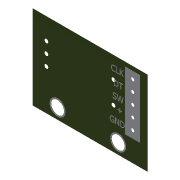
# Autodesk Inventor part: decal_encoder
Saved by Autodesk Inventor 2014 (Build 180170000, 170)
## iProperties
Created: 2015-11-19
Part Number: decal_encoder
Material: Generic
Document SubType Name: Modeling
Designer: Tom
Density: 1 g/cm^3
Appearance: Default
Autodesk Inventor part; units mm, degrees
ref_plane "YZ Plane" through (0, 0, 0) normal (1, 0, 0) x (0, 1, 0)
ref_plane "XZ Plane" through (0, 0, 0) normal (0, 1, 0) x (-1, 0, 0)
ref_plane "XY Plane" through (0, 0, 0) normal (0, 0, 1) x (1, 0, 0)
sketch "0" plane through (0, 0, 0) normal (0, 0, 1) x (1, 0, 0)
  line L0 (0, 0) -> (26.416, 0)
  line L1 (26.416, 0) -> (26.416, 19.3294)
  line L2 (26.416, 19.3294) -> (0, 19.3294)
  line L3 (0, 19.3294) -> (0, 0)
  circle A0 centre (3.175, 14.4018) radius 0.4445
  circle A1 centre (3.175, 11.8618) radius 0.4445
  circle A2 centre (3.175, 9.3218) radius 0.4445
  circle A3 centre (5.7658, 2.4638) radius 1.5
  circle A4 centre (19.685, 2.4638) radius 1.5
  circle A5 centre (23.0251, 6.5532) radius 0.381
  circle A6 centre (23.0251, 9.0932) radius 0.381
  circle A7 centre (23.0251, 11.6332) radius 0.381
  circle A8 centre (23.0251, 14.1732) radius 0.381
  circle A9 centre (23.0251, 16.7132) radius 0.381
  circle A10 centre (5.7658, 2.4638) radius 1.778
  circle A11 centre (19.685, 2.4638) radius 1.778
  line L4 (21.3741, 4.9022) -> (24.6761, 4.9022)
  line L5 (24.6761, 4.9022) -> (24.6761, 18.3642)
  line L6 (21.3741, 18.3642) -> (21.3741, 4.9022)
  circle A12 centre (23.0251, 16.7132) radius 0.4445 projected
  line L7 (24.6761, 18.3642) -> (21.3741, 18.3642)
  line L8 (18.8514, 15.1638) -> (18.8514, 13.6398) projected
  circle A13 centre (18.593, 14.4018) radius 0.4445 projected
  circle A14 centre (18.593, 9.3218) radius 0.4445 projected
  dimension "d0" = 3.556
  dimension "d1" = 3.556
  dimension "d3" = 13.462
  dimension "d4" = 10.16
  dimension "d5" = 13.462
  dimension "d7" = 2.54
  dimension "d8" = 2.54
  dimension "d9" = 2.54
  dimension "d10" = 2.54
  dimension "d11" = 1.651
  dimension "d26" = 0
  dimension "d27" = 2.54
  dimension "d28" = 2.54
  constraints: 16 end point, 12 centre point, 3 vertical alignment, 2 coincident, 2 perpendicular, 1 horizontal, 1 parallel
  measures "d0" diameter of A11
  measures "d1" diameter of A10
  measures "d3" distance of L6.start L4.start
  measures "d4" distance of A5.centre A9.centre
  measures "d5" distance of L5.end L4.end
  measures "d7" distance of A8.centre A9.centre
  measures "d8" distance of A7.centre A8.centre
  measures "d9" distance of A7.centre A6.centre
  measures "d10" distance of A5.centre A6.centre
  measures "d11" horizontal distance of L5.end A9.centre
  measures "d26" vertical distance of A0.centre A13.centre
  measures "d27" distance of A0.centre A1.centre
  measures "d28" distance of A2.centre A1.centre
extrude "Extrusion1" add sketch "0" along normal blind 0.0254 contours L3 L2 L1 L0 | A10 | A11 | L6 L7 L5 L4 | A12 | A13 L8 | L8 A13 | A14
sketch "Sketch3" plane through (0, 0, 0.0254) normal (0, 0, 1) x (1, 0, 0)
  circle A0 centre (23.0251, 16.7132) radius 0.381 projected
  circle A1 centre (23.0251, 14.1732) radius 0.381 projected
  circle A2 centre (23.0251, 11.6332) radius 0.381 projected
  circle A3 centre (23.0251, 9.0932) radius 0.381 projected
  circle A4 centre (23.0251, 6.5532) radius 0.381 projected
  circle A5 centre (19.685, 2.4638) radius 1.5 projected
  circle A6 centre (5.7658, 2.4638) radius 1.5 projected
  line L0 (21.3106, 18.3642) -> (24.7396, 18.3642)
  line L1 (24.7396, 18.3642) -> (24.7396, 4.9022)
  line L2 (24.7396, 4.9022) -> (21.3106, 4.9022)
  line L3 (21.3106, 4.9022) -> (21.3106, 18.3642)
  circle A7 centre (19.685, 2.4638) radius 1.8143
  circle A8 centre (5.7658, 2.4638) radius 1.8161
  line L4 (18.02, 17.393) -> (20.1128, 17.393) construction
  line L5 (20.1128, 17.393) -> (20.1128, 15.9127) construction
  line L6 (20.1128, 15.9127) -> (18.02, 15.9127) construction
  line L7 (18.02, 15.9127) -> (18.02, 17.393) construction
  line L8 (18.6153, 14.6193) -> (20.8208, 14.6193) construction
  line L9 (20.8208, 14.6193) -> (20.8208, 13.19) construction
  line L10 (20.8208, 13.19) -> (18.6153, 13.19) construction
  line L11 (18.6153, 13.19) -> (18.6153, 14.6193) construction
  line L12 (18.3939, 11.9822) -> (20.9411, 11.9822) construction
  line L13 (20.9411, 11.9822) -> (20.9411, 10.6669) construction
  line L14 (20.9411, 10.6669) -> (18.3939, 10.6669) construction
  line L15 (18.3939, 10.6669) -> (18.3939, 11.9822) construction
  line L16 (19.4486, 9.4797) -> (20.7196, 9.4797) construction
  line L17 (20.7196, 9.4797) -> (20.7196, 8.4824) construction
  line L18 (20.7196, 8.4824) -> (19.4486, 8.4824) construction
  line L19 (19.4486, 8.4824) -> (19.4486, 9.4797) construction
  line L20 (17.713, 7.1316) -> (21.2297, 7.1316) construction
  line L21 (21.2297, 7.1316) -> (21.2297, 5.8142) construction
  line L22 (21.2297, 5.8142) -> (17.713, 5.8142) construction
  line L23 (17.713, 5.8142) -> (17.713, 7.1316) construction
  spline S0 degree 2 poles (18.3738, 5.8142) (18.2389, 5.8142) (18.0156, 5.8966) (17.9353, 5.9799) knots 0 0 0 1 2 2 2
  spline S1 degree 2 poles (17.9353, 5.9799) (17.8551, 6.0643) (17.7696, 6.3134) (17.7696, 6.475) knots 0 0 0 1 2 2 2
  spline S2 degree 2 poles (17.7696, 6.475) (17.7696, 6.6283) (17.8561, 6.8712) (17.9364, 6.9576) knots 0 0 0 1 2 2 2
  spline S3 degree 2 poles (17.9364, 6.9576) (18.0135, 7.041) (18.24, 7.1316) (18.3748, 7.1316) knots 0 0 0 1 2 2 2
  spline S4 degree 2 poles (18.3748, 7.1316) (18.4396, 7.1316) (18.557, 7.113) (18.6105, 7.0966) knots 0 0 0 1 2 2 2
  spline S5 degree 2 poles (18.6105, 7.0966) (18.6537, 7.0842) (18.7587, 7.0389) (18.7906, 7.0225) knots 0 0 0 1 2 2 2
  line L24 (18.7906, 7.0225) -> (18.7906, 6.8187)
  line L25 (18.7906, 6.8187) -> (18.7762, 6.8187)
  spline S6 degree 2 poles (18.7762, 6.8187) (18.7443, 6.8465) (18.6774, 6.8969) (18.6156, 6.9257) knots 0 0 0 1 2 2 2
  spline S7 degree 2 poles (18.6156, 6.9257) (18.5642, 6.9515) (18.4314, 6.9854) (18.3552, 6.9854) knots 0 0 0 1 2 2 2
  spline S8 degree 2 poles (18.3552, 6.9854) (18.172, 6.9854) (17.9456, 6.7096) (17.9456, 6.4801) knots 0 0 0 1 2 2 2
  spline S9 degree 2 poles (17.9456, 6.4801) (17.9456, 6.3525) (18.0053, 6.1611) (18.0619, 6.0952) knots 0 0 0 1 2 2 2
  spline S10 degree 2 poles (18.0619, 6.0952) (18.1165, 6.0293) (18.2708, 5.9604) (18.3676, 5.9604) knots 0 0 0 1 2 2 2
  spline S11 degree 2 poles (18.3676, 5.9604) (18.4386, 5.9604) (18.5806, 5.981) (18.629, 6.0015) knots 0 0 0 1 2 2 2
  line L26 (18.629, 6.0015) -> (18.629, 6.3298)
  line L27 (18.629, 6.3298) -> (18.3347, 6.3298)
  line L28 (18.3347, 6.3298) -> (18.3347, 6.478)
  line L29 (18.3347, 6.478) -> (18.7957, 6.478)
  line L30 (18.7957, 6.478) -> (18.7957, 5.9233)
  spline S12 degree 2 poles (18.7957, 5.9233) (18.7638, 5.9089) (18.6547, 5.8647) (18.6084, 5.8513) knots 0 0 0 1 2 2 2
  spline S13 degree 2 poles (18.6084, 5.8513) (18.5456, 5.8328) (18.4448, 5.8142) (18.3738, 5.8142) knots 0 0 0 1 2 2 2
  line L31 (19.9165, 5.8389) -> (19.7271, 5.8389)
  line L32 (19.7271, 5.8389) -> (19.1652, 6.934)
  line L33 (19.1652, 6.934) -> (19.1652, 5.8389)
  line L34 (19.1652, 5.8389) -> (19.0077, 5.8389)
  line L35 (19.0077, 5.8389) -> (19.0077, 7.1089)
  line L36 (19.0077, 7.1089) -> (19.2475, 7.1089)
  line L37 (19.2475, 7.1089) -> (19.759, 6.1034)
  line L38 (19.759, 6.1034) -> (19.759, 7.1089)
  line L39 (19.759, 7.1089) -> (19.9165, 7.1089)
  line L40 (19.9165, 7.1089) -> (19.9165, 5.8389)
  spline S14 degree 2 poles (21.1752, 6.4729) (21.1752, 6.299) (21.0342, 6.019) (20.9158, 5.9408) knots 0 0 0 1 2 2 2
  spline S15 degree 2 poles (20.9158, 5.9408) (20.8191, 5.8801) (20.6204, 5.8389) (20.4661, 5.8389) knots 0 0 0 1 2 2 2
  line L41 (20.4661, 5.8389) -> (20.1738, 5.8389)
  line L42 (20.1738, 5.8389) -> (20.1738, 7.1089)
  line L43 (20.1738, 7.1089) -> (20.463, 7.1089)
  spline S16 degree 2 poles (20.463, 7.1089) (20.6421, 7.1089) (20.8458, 7.0554) (20.9179, 7.0081) knots 0 0 0 1 2 2 2
  spline S17 degree 2 poles (20.9179, 7.0081) (21.0403, 6.9268) (21.1752, 6.6582) (21.1752, 6.4729) knots 0 0 0 1 2 2 2
  spline S18 degree 2 poles (20.9992, 6.475) (20.9992, 6.6211) (20.9024, 6.828) (20.8067, 6.8866) knots 0 0 0 1 2 2 2
  spline S19 degree 2 poles (20.8067, 6.8866) (20.7388, 6.9268) (20.5855, 6.9628) (20.4712, 6.9628) knots 0 0 0 1 2 2 2
  line L44 (20.4712, 6.9628) -> (20.3426, 6.9628)
  line L45 (20.3426, 6.9628) -> (20.3426, 5.9851)
  line L46 (20.3426, 5.9851) -> (20.4712, 5.9851)
  spline S20 degree 2 poles (20.4712, 5.9851) (20.5834, 5.9851) (20.7532, 6.0211) (20.8222, 6.0695) knots 0 0 0 1 2 2 2
  spline S21 degree 2 poles (20.8222, 6.0695) (20.9107, 6.1292) (20.9992, 6.3268) (20.9992, 6.475) knots 0 0 0 1 2 2 2
  line L47 (20.5858, 8.9126) -> (20.1556, 8.9126)
  line L48 (20.1556, 8.9126) -> (20.1556, 8.4824)
  line L49 (20.1556, 8.4824) -> (20.0136, 8.4824)
  line L50 (20.0136, 8.4824) -> (20.0136, 8.9126)
  line L51 (20.0136, 8.9126) -> (19.5834, 8.9126)
  line L52 (19.5834, 8.9126) -> (19.5834, 9.0495)
  line L53 (19.5834, 9.0495) -> (20.0136, 9.0495)
  line L54 (20.0136, 9.0495) -> (20.0136, 9.4797)
  line L55 (20.0136, 9.4797) -> (20.1556, 9.4797)
  line L56 (20.1556, 9.4797) -> (20.1556, 9.0495)
  line L57 (20.1556, 9.0495) -> (20.5858, 9.0495)
  line L58 (20.5858, 9.0495) -> (20.5858, 8.9126)
  spline S22 degree 2 poles (18.8765, 10.6669) (18.7386, 10.6669) (18.5451, 10.7245) (18.4597, 10.7657) knots 0 0 0 1 2 2 2
  line L59 (18.4597, 10.7657) -> (18.4597, 10.9777)
  line L60 (18.4597, 10.9777) -> (18.4721, 10.9777)
  spline S23 degree 2 poles (18.4721, 10.9777) (18.5554, 10.8995) (18.7664, 10.813) (18.8642, 10.813) knots 0 0 0 1 2 2 2
  spline S24 degree 2 poles (18.8642, 10.813) (19.0042, 10.813) (19.1472, 10.9293) (19.1472, 11.0251) knots 0 0 0 1 2 2 2
  spline S25 degree 2 poles (19.1472, 11.0251) (19.1472, 11.1012) (19.0721, 11.1959) (18.9908, 11.2196) knots 0 0 0 1 2 2 2
  spline S26 degree 2 poles (18.9908, 11.2196) (18.9321, 11.236) (18.8343, 11.2587) (18.7613, 11.2772) knots 0 0 0 1 2 2 2
  spline S27 degree 2 poles (18.7613, 11.2772) (18.6954, 11.2947) (18.5915, 11.3472) (18.5513, 11.3894) knots 0 0 0 1 2 2 2
  spline S28 degree 2 poles (18.5513, 11.3894) (18.5122, 11.4316) (18.469, 11.5448) (18.469, 11.6189) knots 0 0 0 1 2 2 2
  spline S29 degree 2 poles (18.469, 11.6189) (18.469, 11.7733) (18.7098, 11.9822) (18.8961, 11.9822) knots 0 0 0 1 2 2 2
  spline S30 degree 2 poles (18.8961, 11.9822) (19.0031, 11.9822) (19.1925, 11.94) (19.2738, 11.8999) knots 0 0 0 1 2 2 2
  line L61 (19.2738, 11.8999) -> (19.2738, 11.6981)
  line L62 (19.2738, 11.6981) -> (19.2614, 11.6981)
  spline S31 degree 2 poles (19.2614, 11.6981) (19.2007, 11.7537) (19.0114, 11.836) (18.9074, 11.836) knots 0 0 0 1 2 2 2
  spline S32 degree 2 poles (18.9074, 11.836) (18.7901, 11.836) (18.645, 11.7259) (18.645, 11.6364) knots 0 0 0 1 2 2 2
  spline S33 degree 2 poles (18.645, 11.6364) (18.645, 11.5561) (18.7304, 11.4604) (18.8107, 11.4388) knots 0 0 0 1 2 2 2
  spline S34 degree 2 poles (18.8107, 11.4388) (18.8642, 11.4244) (19.0196, 11.3873) (19.071, 11.3719) knots 0 0 0 1 2 2 2
  spline S35 degree 2 poles (19.071, 11.3719) (19.2018, 11.3317) (19.3232, 11.1702) (19.3232, 11.0518) knots 0 0 0 1 2 2 2
  spline S36 degree 2 poles (19.3232, 11.0518) (19.3232, 10.9767) (19.2625, 10.8326) (19.2079, 10.7822) knots 0 0 0 1 2 2 2
  spline S37 degree 2 poles (19.2079, 10.7822) (19.1472, 10.7266) (18.9928, 10.6669) (18.8765, 10.6669) knots 0 0 0 1 2 2 2
  line L63 (20.9184, 11.9595) -> (20.5994, 10.6895)
  line L64 (20.5994, 10.6895) -> (20.41, 10.6895)
  line L65 (20.41, 10.6895) -> (20.1517, 11.7434)
  line L66 (20.1517, 11.7434) -> (19.9006, 10.6895)
  line L67 (19.9006, 10.6895) -> (19.7133, 10.6895)
  line L68 (19.7133, 10.6895) -> (19.3891, 11.9595)
  line L69 (19.3891, 11.9595) -> (19.563, 11.9595)
  line L70 (19.563, 11.9595) -> (19.8182, 10.9067)
  line L71 (19.8182, 10.9067) -> (20.0714, 11.9595)
  line L72 (20.0714, 11.9595) -> (20.2433, 11.9595)
  line L73 (20.2433, 11.9595) -> (20.4985, 10.8944)
  line L74 (20.4985, 10.8944) -> (20.7527, 11.9595)
  line L75 (20.7527, 11.9595) -> (20.9184, 11.9595)
  spline S38 degree 2 poles (19.7453, 13.9833) (19.7453, 13.8093) (19.6043, 13.5294) (19.4859, 13.4512) knots 0 0 0 1 2 2 2
  spline S39 degree 2 poles (19.4859, 13.4512) (19.3892, 13.3905) (19.1906, 13.3493) (19.0362, 13.3493) knots 0 0 0 1 2 2 2
  line L76 (19.0362, 13.3493) -> (18.7439, 13.3493)
  line L77 (18.7439, 13.3493) -> (18.7439, 14.6193)
  line L78 (18.7439, 14.6193) -> (19.0331, 14.6193)
  spline S40 degree 2 poles (19.0331, 14.6193) (19.2122, 14.6193) (19.416, 14.5658) (19.488, 14.5184) knots 0 0 0 1 2 2 2
  spline S41 degree 2 poles (19.488, 14.5184) (19.6105, 14.4371) (19.7453, 14.1685) (19.7453, 13.9833) knots 0 0 0 1 2 2 2
  spline S42 degree 2 poles (19.5693, 13.9853) (19.5693, 14.1315) (19.4726, 14.3383) (19.3769, 14.397) knots 0 0 0 1 2 2 2
  spline S43 degree 2 poles (19.3769, 14.397) (19.3089, 14.4371) (19.1556, 14.4732) (19.0413, 14.4732) knots 0 0 0 1 2 2 2
  line L79 (19.0413, 14.4732) -> (18.9127, 14.4732)
  line L80 (18.9127, 14.4732) -> (18.9127, 13.4954)
  line L81 (18.9127, 13.4954) -> (19.0413, 13.4954)
  spline S44 degree 2 poles (19.0413, 13.4954) (19.1535, 13.4954) (19.3233, 13.5315) (19.3923, 13.5798) knots 0 0 0 1 2 2 2
  spline S45 degree 2 poles (19.3923, 13.5798) (19.4808, 13.6395) (19.5693, 13.8371) (19.5693, 13.9853) knots 0 0 0 1 2 2 2
  line L82 (20.2249, 13.3493) -> (20.2249, 14.469)
  line L83 (20.2249, 14.469) -> (19.7988, 14.469)
  line L84 (19.7988, 14.469) -> (19.7988, 14.6193)
  line L85 (19.7988, 14.6193) -> (20.8198, 14.6193)
  line L86 (20.8198, 14.6193) -> (20.8198, 14.469)
  line L87 (20.8198, 14.469) -> (20.3937, 14.469)
  line L88 (20.3937, 14.469) -> (20.3937, 13.3493)
  line L89 (20.3937, 13.3493) -> (20.2249, 13.3493)
  spline S46 degree 2 poles (18.6447, 16.0777) (18.5212, 16.0777) (18.3122, 16.1611) (18.2361, 16.2444) knots 0 0 0 1 2 2 2
  spline S47 degree 2 poles (18.2361, 16.2444) (18.1599, 16.3268) (18.0766, 16.5738) (18.0766, 16.7343) knots 0 0 0 1 2 2 2
  spline S48 degree 2 poles (18.0766, 16.7343) (18.0766, 16.8938) (18.1579, 17.1305) (18.2351, 17.218) knots 0 0 0 1 2 2 2
  spline S49 degree 2 poles (18.2351, 17.218) (18.3112, 17.3034) (18.5191, 17.393) (18.6478, 17.393) knots 0 0 0 1 2 2 2
  spline S50 degree 2 poles (18.6478, 17.393) (18.7116, 17.393) (18.8237, 17.3745) (18.8711, 17.36) knots 0 0 0 1 2 2 2
  spline S51 degree 2 poles (18.8711, 17.36) (18.9123, 17.3467) (18.9977, 17.3086) (19.0399, 17.2859) knots 0 0 0 1 2 2 2
  line L90 (19.0399, 17.2859) -> (19.0399, 17.0822)
  line L91 (19.0399, 17.0822) -> (19.0265, 17.0822)
  spline S52 degree 2 poles (19.0265, 17.0822) (19.0039, 17.1028) (18.9339, 17.1604) (18.8834, 17.1882) knots 0 0 0 1 2 2 2
  spline S53 degree 2 poles (18.8834, 17.1882) (18.8351, 17.2149) (18.7208, 17.2489) (18.6467, 17.2489) knots 0 0 0 1 2 2 2
  spline S54 degree 2 poles (18.6467, 17.2489) (18.5654, 17.2489) (18.4203, 17.182) (18.3658, 17.1182) knots 0 0 0 1 2 2 2
  spline S55 degree 2 poles (18.3658, 17.1182) (18.3122, 17.0534) (18.2526, 16.8568) (18.2526, 16.7343) knots 0 0 0 1 2 2 2
  spline S56 degree 2 poles (18.2526, 16.7343) (18.2526, 16.6036) (18.3153, 16.4153) (18.3699, 16.3504) knots 0 0 0 1 2 2 2
  spline S57 degree 2 poles (18.3699, 16.3504) (18.4234, 16.2876) (18.5665, 16.2238) (18.6467, 16.2238) knots 0 0 0 1 2 2 2
  spline S58 degree 2 poles (18.6467, 16.2238) (18.7198, 16.2238) (18.8443, 16.2599) (18.8927, 16.2866) knots 0 0 0 1 2 2 2
  spline S59 degree 2 poles (18.8927, 16.2866) (18.939, 16.3134) (19.008, 16.369) (19.0275, 16.3885) knots 0 0 0 1 2 2 2
  line L92 (19.0275, 16.3885) -> (19.0399, 16.3885)
  line L93 (19.0399, 16.3885) -> (19.0399, 16.1868)
  spline S60 degree 2 poles (19.0399, 16.1868) (18.9977, 16.1672) (18.9236, 16.1312) (18.8711, 16.1147) knots 0 0 0 1 2 2 2
  spline S61 degree 2 poles (18.8711, 16.1147) (18.8155, 16.0962) (18.7208, 16.0777) (18.6447, 16.0777) knots 0 0 0 1 2 2 2
  line L94 (19.9332, 16.1003) -> (19.1973, 16.1003)
  line L95 (19.1973, 16.1003) -> (19.1973, 17.3703)
  line L96 (19.1973, 17.3703) -> (19.3661, 17.3703)
  line L97 (19.3661, 17.3703) -> (19.3661, 16.2506)
  line L98 (19.3661, 16.2506) -> (19.9332, 16.2506)
  line L99 (19.9332, 16.2506) -> (19.9332, 16.1003)
  line L100 (20.9922, 16.1003) -> (20.773, 16.1003)
  line L101 (20.773, 16.1003) -> (20.3088, 16.6911)
  line L102 (20.3088, 16.6911) -> (20.2347, 16.6077)
  line L103 (20.2347, 16.6077) -> (20.2347, 16.1003)
  line L104 (20.2347, 16.1003) -> (20.066, 16.1003)
  line L105 (20.066, 16.1003) -> (20.066, 17.3703)
  line L106 (20.066, 17.3703) -> (20.2347, 17.3703)
  line L107 (20.2347, 17.3703) -> (20.2347, 16.7868)
  line L108 (20.2347, 16.7868) -> (20.7555, 17.3703)
  line L109 (20.7555, 17.3703) -> (20.9613, 17.3703)
  line L110 (20.9613, 17.3703) -> (20.4354, 16.8033)
  line L111 (20.4354, 16.8033) -> (20.9922, 16.1003)
  dimension "d3" = 13.462
  dimension "d4" = 10.16
  dimension "d5" = 13.462
  dimension "d7" = 2.54
  dimension "d8" = 2.54
  dimension "d9" = 2.54
  dimension "d10" = 2.54
  dimension "d11" = 1.651
  dimension "d14" = 3.429
  dimension "d15" = 13.462
  dimension "d16" = 1.7145
  dimension "d17" = 1.651
  dimension "d18" = 10.16
  dimension "d19" = 3.6322
  constraints: 8 end point, 2 centre point, 2 coincident, 2 parallel, 1 horizontal, 1 perpendicular, 10 other
  measures "d14" distance of L0.start L0.end
  measures "d15" distance of L0.end L1.end
  measures "d16" distance from line of L1 A0.centre
  measures "d17" distance from line of L0 A0.centre
  measures "d18" distance of A0.centre A4.centre
  measures "d19" diameter of A8
extrude "Extrusion2" add sketch "Sketch3" along normal blind 0.0254
sketch "Sketch4" plane through (0, 0, 0.0254) normal (0, 0, 1) x (1, 0, 0)
  line L0 (18.4704, 9.7028) -> (18.4704, 8.9408) projected
  line L1 (18.4704, 14.7828) -> (18.4704, 14.0208) projected
  line L2 (18.3347, 14.4018) -> (18.8514, 14.4018)
  line L3 (18.3347, 9.3218) -> (18.8514, 9.3218)
  line L4 (18.8514, 9.7028) -> (18.8514, 8.9408) projected
  line L5 (18.8514, 14.7828) -> (18.8514, 14.0208) projected
  circle A0 centre (18.593, 9.3218) radius 0.4445
  circle A1 centre (18.593, 14.4018) radius 0.4445
  dimension "d22" = 0.889
  dimension "d23" = 0.889
  constraints: 4 end point, 4 midpoint, 2 centre point, 1 parallel, 1 perpendicular
  measures "d22" diameter of A0
  measures "d23" diameter of A1
extrude "Extrusion3" cut sketch "Sketch4" against normal through all
equation "\"d11\" = 0.5 * d2"
equation "\"d16\" = 0.5 * d14"
equation "\"d2\" = 3.302"
body "Solid1"
